nixal_reprap4040_XtensionerHolder (Autodesk Fusion 360 design; units mm, degrees)
Autodesk Fusion 360 part; units mm, degrees
sketch "Sketch1" plane through (0, 0, 0) normal (0, 1, 0) x (1, 0, 0)
  line L0 (0, 0) -> (8.3, 0)
  line L1 (8.3, 0) -> (8.3, 24.7)
  line L2 (8.3, 24.7) -> (0, 24.7)
  line L3 (0, 24.7) -> (0, 0)
  line L4 (-4, 26.2) -> (12.3, 26.2)
  line L5 (12.3, 26.2) -> (12.3, -1.5)
  line L6 (12.3, -1.5) -> (-4, -1.5)
  line L7 (-4, -1.5) -> (-4, 26.2)
  line L8 (0, 24.7) -> (8.3, 0) construction
  line L9 (8.3, 24.7) -> (0, 0) construction
  circle A0 centre (4.15, 12.35) radius 1.65
  line L10 (7.4, 9.1) -> (0.9, 15.6) construction
  line L11 (0.9, 9.1) -> (7.4, 15.6) construction
  circle A1 centre (4.15, 12.35) radius 3.25
  dimension "d1" = 24.7
  dimension "d2" = 8.3
  dimension "d3" = 4
  dimension "d4" = 4
  dimension "d5" = 1.5
  dimension "d6" = 1.5
  dimension "d7" = 3.3
  dimension "d15" = 6.5
  constraint horizontal L0
  constraint vertical L1
  constraint horizontal L2
  constraint vertical L3
  constraint coincident L0.start L3.end
  constraint horizontal L4
  constraint vertical L5
  constraint horizontal L6
  constraint vertical L7
  constraint midpoint L9
  constraint coincident L10
  constraint coincident L11
  measures "d1" distance of L0.start
  measures "d3" distance of L1 L5
  measures "d4" distance of L3 L7
  measures "d5" distance of L2 L4
  measures "d6" distance of L0 L6
  measures "d7" diameter of A0
  measures "d15" diameter of A1
extrude "Extrude1" add sketch "Sketch1" along normal blind 3 contours L0 L1 L2 L3 | L4 L5 L6 L7 | A1 makes body 1
extrude "Extrude2" add sketch "Sketch1" along normal blind 10 and the other way blind -3 separate body contours L0 L1 L2 L3 | A1 makes body 2
extrude "Extrude3" cut sketch "Sketch1" along normal blind 6 contours A1 bodies 1 2
